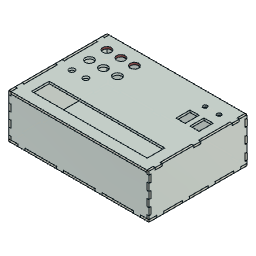
SimDash_Fusion (Autodesk Fusion 360 design; units mm, degrees)
Autodesk Fusion 360 part; units mm, degrees
(part 1 of 2)
sketch "Skizze1" plane through (0, 0, 0) normal (0, 0, 1) x (1, 0, 0)
  line L0 (-100, 70) -> (100, 70)
  line L1 (100, 70) -> (100, -70)
  line L2 (100, -70) -> (-100, -70)
  line L3 (-100, -70) -> (-100, 70)
  line L4 (-100, 70) -> (100, -70) construction
  line L5 (100, 70) -> (-100, -70) construction
  dimension "d1" = 200
  dimension "d2" = 140
  constraint horizontal L0
  constraint perpendicular L0 L1
  constraint parallel L0 L2
  constraint parallel L1 L3
  constraint coincident L4 origin
  constraint coincident L5 origin
  measures "d1" distance of L1.end L2.end
  measures "d2" distance of L0.end L1.end
extrude "Extrusion1" add sketch "Skizze1" along normal blind 3 makes body 1
sketch "Skizze2" plane through (0, 0, 3) normal (0, 0, 1) x (-1, 0, 0)
  line L0 (100, 70) -> (-100, 70)
  line L1 (-100, 70) -> (-100, -70)
  line L2 (-100, -70) -> (100, -70)
  line L3 (100, -70) -> (100, 70)
  line L4 (100, -70) -> (97, -70)
  line L5 (97, -70) -> (97, 70)
  line L6 (97, 70) -> (100, 70)
  line L7 (100, 70) -> (100, -70)
  dimension "d5" = 3
  constraint horizontal L4
  constraint vertical L5
  constraint horizontal L6
  constraint vertical L7
  constraint coincident L2.end L3.start
  measures "d5" distance of L2.end L4.end
extrude "Extrusion2" add sketch "Skizze2" along normal blind 60 separate body contours L0 L2 L3 L4 L5 L6 L7 picked at (99, 23.333333) makes body 2
sketch "Skizze3" plane through (0, 0, 3) normal (0, 0, -1) x (1, 0, 0)
  line L0 (-97, 70) -> (-100, 70)
  line L1 (-100, 70) -> (-100, -70)
  line L2 (-100, -70) -> (-97, -70)
  line L3 (-97, -70) -> (-97, 70)
  line L4 (-100, 60) -> (-97, 60)
  line L5 (-97, 60) -> (-97, 50)
  line L6 (-97, 50) -> (-100, 50)
  line L7 (-100, 50) -> (-100, 60)
  dimension "d8" = 3
  dimension "d9" = 10
  constraint horizontal L4
  constraint vertical L5
  constraint horizontal L6
  constraint vertical L7
  constraint coincident L1 L4.start
  measures "d8" distance of L4.start L4.end
  measures "d9" distance of L4.start L6.end
extrude "Extrusion3" add sketch "Skizze3" along normal blind 3 contours L1 L3 L4 L5 L6 L7 picked at (-99, 56.666667) bodies 2
pattern_linear "R-Anordnung1" count 4 spacing 36.666667 along (0, 1, 0) of "Extrusion3"
combine "Kombinieren1" operation cut target body 1 tool bodies 2 keep tools
sketch "Skizze4" plane through (0, 0, 3) normal (0, 0, 1) x (-1, 0, 0)
  line L0 (97, -60) -> (97, -50)
  line L1 (97, -50) -> (100, -50)
  line L2 (100, -50) -> (100, -23.333333)
  line L3 (100, -23.333333) -> (97, -23.333333)
  line L4 (97, -23.333333) -> (97, -13.333333)
  line L5 (97, -13.333333) -> (100, -13.333333)
  line L6 (100, -13.333333) -> (100, 13.333333)
  line L7 (100, 13.333333) -> (97, 13.333333)
  line L8 (97, 13.333333) -> (97, 23.333333)
  line L9 (97, 23.333333) -> (100, 23.333333)
  line L10 (100, 23.333333) -> (100, 50)
  line L11 (100, 50) -> (97, 50)
  line L12 (97, 50) -> (97, 60)
  line L13 (97, 60) -> (100, 60)
  line L14 (100, 60) -> (100, 70)
  line L15 (100, 70) -> (-100, 70)
  line L16 (-100, 70) -> (-100, -70)
  line L17 (-100, -70) -> (100, -70)
  line L18 (100, -70) -> (100, -60)
  line L19 (100, -60) -> (97, -60)
  line L20 (-100, -70) -> (-97, -70)
  line L21 (-97, -70) -> (-97, 70)
  line L22 (-97, 70) -> (-100, 70)
  line L23 (-100, 70) -> (-100, -70)
  dimension "d16" = 3
  constraint horizontal L20
  constraint vertical L21
  constraint horizontal L22
  constraint vertical L23
  constraint coincident L16.end L17.start
  measures "d16" distance of L16.end L20.end
sketch "Skizze6" plane through (0, 0, 3) normal (0, 0, 1) x (-1, 0, 0)
  line L0 (-100, -70) -> (100, -70)
  line L1 (100, -70) -> (100, -60)
  line L2 (100, -60) -> (97, -60)
  line L3 (97, -60) -> (97, -50)
  line L4 (97, -50) -> (100, -50)
  line L5 (100, -50) -> (100, -23.333333)
  line L6 (100, -23.333333) -> (97, -23.333333)
  line L7 (97, -23.333333) -> (97, -13.333333)
  line L8 (97, -13.333333) -> (100, -13.333333)
  line L9 (100, -13.333333) -> (100, 13.333333)
  line L10 (100, 13.333333) -> (97, 13.333333)
  line L11 (97, 13.333333) -> (97, 23.333333)
  line L12 (97, 23.333333) -> (100, 23.333333)
  line L13 (100, 23.333333) -> (100, 50)
  line L14 (100, 50) -> (97, 50)
  line L15 (97, 50) -> (97, 60)
  line L16 (97, 60) -> (100, 60)
  line L17 (100, 60) -> (100, 70)
  line L18 (100, 70) -> (-100, 70)
  line L19 (-100, 70) -> (-100, -70)
  line L20 (97.000041, -70) -> (-96.999959, -70)
  line L21 (-96.999959, -70) -> (-96.999959, -67)
  line L22 (-96.999959, -67) -> (97.000041, -67)
  line L23 (97.000041, -67) -> (97.000041, -70)
  dimension "d26" = 194
  dimension "d27" = 3
  constraint horizontal L20
  constraint vertical L21
  constraint horizontal L22
  constraint vertical L23
extrude "Extrusion6" add sketch "Skizze6" along normal blind 60 separate body contours L0 L20 L21 L22 L23 picked at (-32.333293, -68) makes body 3
sketch "Skizze7" plane through (96.999959, 0, 0) normal (1, 0, 0) x (0, 1, 0)
  line L0 (67, 3) -> (70, 3)
  line L1 (70, 3) -> (70, 63)
  line L2 (70, 63) -> (67, 63)
  line L3 (67, 63) -> (67, 3)
  line L4 (67, 58.682652) -> (70, 58.682652)
  line L5 (70, 58.682652) -> (70, 48.682652)
  line L6 (70, 48.682652) -> (67, 48.682652)
  line L7 (67, 48.682652) -> (67, 58.682652)
  dimension "d30" = 10
  constraint horizontal L4
  constraint vertical L5
  constraint horizontal L6
  constraint vertical L7
extrude "Extrusion7" add sketch "Skizze7" along normal blind 3.1 contours L1 L3 L4 L5 L6 L7 picked at (68, 55.349319) bodies 3
pattern_linear "R-Anordnung3" count 3 spacing 21 along (0, 0, -1) of "Extrusion7"
sketch "Skizze10" plane through (-97.000041, 0, 0) normal (-1, 0, 0) x (0, -1, 0)
  line L0 (-70, 3) -> (-67, 3)
  line L1 (-67, 3) -> (-67, 63)
  line L2 (-67, 63) -> (-70, 63)
  line L3 (-70, 63) -> (-70, 3)
  line L4 (-70, 58.048511) -> (-67, 58.048511)
  line L5 (-67, 58.048511) -> (-67, 48.048511)
  line L6 (-67, 48.048511) -> (-70, 48.048511)
  line L7 (-70, 48.048511) -> (-70, 58.048511)
  dimension "d43" = 10
  constraint horizontal L4
  constraint vertical L5
  constraint horizontal L6
  constraint vertical L7
extrude "Extrusion10" add sketch "Skizze10" along normal blind 3 contours L1 L3 L4 L5 L6 L7 picked at (-69, 54.715177) bodies 3
pattern_linear "R-Anordnung4" count 3 spacing 20 along (0, 0, -1) of "Extrusion10"
sketch "Skizze11" plane through (0, 0, 3) normal (0, 0, -1) x (1, 0, 0)
  line L0 (96.999959, -67) -> (-97.000041, -67)
  line L1 (-97.000041, -67) -> (-97.000041, -70)
  line L2 (-97.000041, -70) -> (96.999959, -70)
  line L3 (96.999959, -70) -> (96.999959, -67)
  line L4 (-90.254959, -67) -> (-80.254959, -67)
  line L5 (-80.254959, -67) -> (-80.254959, -70)
  line L6 (-80.254959, -70) -> (-90.254959, -70)
  line L7 (-90.254959, -70) -> (-90.254959, -67)
  dimension "d50" = 10
  constraint horizontal L4
  constraint vertical L5
  constraint horizontal L6
  constraint vertical L7
extrude "Extrusion11" add sketch "Skizze11" along normal blind 3 contours L0 L2 L4 L5 L6 L7 picked at (-86.921626, -68) bodies 3
pattern_linear "R-Anordnung5" count 4 spacing 56.666667 along (1, 0, 0) of "Extrusion11"
combine "Kombinieren3" operation cut target body 2 tool bodies 3 keep tools
combine "Kombinieren4" operation cut target body 1 tool bodies 3 keep tools
sketch "Skizze12" plane through (0, 0, 3) normal (0, 0, 1) x (-1, 0, 0)
  line L0 (-100, -70) -> (-89.745041, -70)
  line L1 (-89.745041, -70) -> (-89.745041, -67)
  line L2 (-89.745041, -67) -> (-79.745041, -67)
  line L3 (-79.745041, -67) -> (-79.745041, -70)
  line L4 (-79.745041, -70) -> (-33.078374, -70)
  line L5 (-33.078374, -70) -> (-33.078374, -67)
  line L6 (-33.078374, -67) -> (-23.078374, -67)
  line L7 (-23.078374, -67) -> (-23.078374, -70)
  line L8 (-23.078374, -70) -> (23.588293, -70)
  line L9 (23.588293, -70) -> (23.588293, -67)
  line L10 (23.588293, -67) -> (33.588293, -67)
  line L11 (33.588293, -67) -> (33.588293, -70)
  line L12 (33.588293, -70) -> (80.254959, -70)
  line L13 (80.254959, -70) -> (80.254959, -67)
  line L14 (80.254959, -67) -> (90.254959, -67)
  line L15 (90.254959, -67) -> (90.254959, -70)
  line L16 (90.254959, -70) -> (100, -70)
  line L17 (100, -70) -> (100, -60)
  line L18 (100, -60) -> (97, -60)
  line L19 (97, -60) -> (97, -50)
  line L20 (97, -50) -> (100, -50)
  line L21 (100, -50) -> (100, -23.333333)
  line L22 (100, -23.333333) -> (97, -23.333333)
  line L23 (97, -23.333333) -> (97, -13.333333)
  line L24 (97, -13.333333) -> (100, -13.333333)
  line L25 (100, -13.333333) -> (100, 13.333333)
  line L26 (100, 13.333333) -> (97, 13.333333)
  line L27 (97, 13.333333) -> (97, 23.333333)
  line L28 (97, 23.333333) -> (100, 23.333333)
  line L29 (100, 23.333333) -> (100, 50)
  line L30 (100, 50) -> (97, 50)
  line L31 (97, 50) -> (97, 60)
  line L32 (97, 60) -> (100, 60)
  line L33 (100, 60) -> (100, 70)
  line L34 (100, 70) -> (-100, 70)
  line L35 (-100, 70) -> (-100, -70)
  line L36 (-100, -70) -> (-97, -70)
  line L37 (-97, -70) -> (-97, 70)
  line L38 (-97, 70) -> (-100, 70)
  line L39 (-100, 70) -> (-100, -70)
  dimension "d59" = 3
  constraint horizontal L36
  constraint vertical L37
  constraint horizontal L38
  constraint vertical L39
  constraint coincident L0.start L35.end
  measures "d59" distance of L0.start L36.end
extrude "Extrusion13" add sketch "Skizze12" along normal blind 60 separate body contours L0 L34 L35 L36 L37 L38 L39 picked at (-99, 23.333333) makes body 4
combine "Kombinieren5" operation cut target body 4 tool bodies 3 keep tools
combine "Kombinieren6" operation cut target body 4 tool bodies 3 keep tools
sketch "Skizze13" plane through (0, 0, 3) normal (0, 0, -1) x (1, 0, 0)
  line L0 (100, -70) -> (100, 70)
  line L1 (100, 70) -> (97, 70)
  line L2 (97, 70) -> (97, -70)
  line L3 (97, -70) -> (100, -70)
  line L4 (97, 58.902439) -> (100, 58.902439)
  line L5 (100, 58.902439) -> (100, 48.902439)
  line L6 (100, 48.902439) -> (97, 48.902439)
  line L7 (97, 48.902439) -> (97, 58.902439)
  dimension "d62" = 10
  constraint horizontal L4
  constraint vertical L5
  constraint horizontal L6
  constraint vertical L7
extrude "Extrusion14" add sketch "Skizze13" along normal blind 3 contours L0 L2 L4 L5 L6 L7 picked at (99, 52.235772) bodies 4
pattern_linear "R-Anordnung6" count 4 spacing 36.666667 along (0, 1, 0) of "Extrusion14"
combine "Kombinieren7" operation cut target body 1 tool bodies 4 keep tools
sketch "Skizze14" plane through (0, 0, 3) normal (0, 0, 1) x (-1, 0, 0)
  line L0 (-97, 58.902439) -> (-97, 48.902439)
  line L1 (-97, 48.902439) -> (-100, 48.902439)
  line L2 (-100, 48.902439) -> (-100, 22.235772)
  line L3 (-100, 22.235772) -> (-97, 22.235772)
  line L4 (-97, 22.235772) -> (-97, 12.235772)
  line L5 (-97, 12.235772) -> (-100, 12.235772)
  line L6 (-100, 12.235772) -> (-100, -14.430895)
  line L7 (-100, -14.430895) -> (-97, -14.430895)
  line L8 (-97, -14.430895) -> (-97, -24.430895)
  line L9 (-97, -24.430895) -> (-100, -24.430895)
  line L10 (-100, -24.430895) -> (-100, -51.097561)
  line L11 (-100, -51.097561) -> (-97, -51.097561)
  line L12 (-97, -51.097561) -> (-97, -61.097561)
  line L13 (-97, -61.097561) -> (-100, -61.097561)
  line L14 (-100, -61.097561) -> (-100, -70)
  line L15 (-100, -70) -> (-89.745041, -70)
  line L16 (-89.745041, -70) -> (-89.745041, -67)
  line L17 (-89.745041, -67) -> (-79.745041, -67)
  line L18 (-79.745041, -67) -> (-79.745041, -70)
  line L19 (-79.745041, -70) -> (-33.078374, -70)
  line L20 (-33.078374, -70) -> (-33.078374, -67)
  line L21 (-33.078374, -67) -> (-23.078374, -67)
  line L22 (-23.078374, -67) -> (-23.078374, -70)
  line L23 (-23.078374, -70) -> (23.588293, -70)
  line L24 (23.588293, -70) -> (23.588293, -67)
  line L25 (23.588293, -67) -> (33.588293, -67)
  line L26 (33.588293, -67) -> (33.588293, -70)
  line L27 (33.588293, -70) -> (80.254959, -70)
  line L28 (80.254959, -70) -> (80.254959, -67)
  line L29 (80.254959, -67) -> (90.254959, -67)
  line L30 (90.254959, -67) -> (90.254959, -70)
  line L31 (90.254959, -70) -> (100, -70)
  line L32 (100, -70) -> (100, -60)
  line L33 (100, -60) -> (97, -60)
  line L34 (97, -60) -> (97, -50)
  line L35 (97, -50) -> (100, -50)
  line L36 (100, -50) -> (100, -23.333333)
  line L37 (100, -23.333333) -> (97, -23.333333)
  line L38 (97, -23.333333) -> (97, -13.333333)
  line L39 (97, -13.333333) -> (100, -13.333333)
  line L40 (100, -13.333333) -> (100, 13.333333)
  line L41 (100, 13.333333) -> (97, 13.333333)
  line L42 (97, 13.333333) -> (97, 23.333333)
  line L43 (97, 23.333333) -> (100, 23.333333)
  line L44 (100, 23.333333) -> (100, 50)
  line L45 (100, 50) -> (97, 50)
  line L46 (97, 50) -> (97, 60)
  line L47 (97, 60) -> (100, 60)
  line L48 (100, 60) -> (100, 70)
  line L49 (100, 70) -> (-100, 70)
  line L50 (-100, 70) -> (-100, 58.902439)
  line L51 (-100, 58.902439) -> (-97, 58.902439)
  line L52 (97, 70) -> (-97.000001, 70)
  line L53 (-97.000001, 70) -> (-97.000001, 67)
  line L54 (-97.000001, 67) -> (97, 67)
  line L55 (97, 67) -> (97, 70)
  dimension "d69" = 3
  constraint horizontal L52
  constraint vertical L53
  constraint horizontal L54
  constraint vertical L55
  constraint coincident L49 L52.start
  measures "d69" distance of L52.start L54.end
extrude "Extrusion15" add sketch "Skizze14" along normal blind 60 separate body contours L49 L52 L53 L54 L55 picked at (-32.333334, 69) makes body 5
sketch "Skizze15" plane through (-97, 0, 0) normal (-1, 0, 0) x (0, -1, 0)
  line L0 (67, 3) -> (70, 3)
  line L1 (70, 3) -> (70, 63)
  line L2 (70, 63) -> (67, 63)
  line L3 (67, 63) -> (67, 3)
  line L4 (67, 57.564108) -> (70, 57.564108)
  line L5 (70, 57.564108) -> (70, 47.564108)
  line L6 (70, 47.564108) -> (67, 47.564108)
  line L7 (67, 47.564108) -> (67, 57.564108)
  dimension "d72" = 10
  constraint horizontal L4
  constraint vertical L5
  constraint horizontal L6
  constraint vertical L7
extrude "Extrusion16" add sketch "Skizze15" along normal blind 3 contours L1 L3 L4 L5 L6 L7 picked at (68, 54.230775) bodies 5
pattern_linear "R-Anordnung7" count 3 spacing 20 along (0, 0, -1) of "Extrusion16"
combine "Kombinieren8" operation cut target body 2 tool bodies 5 keep tools
sketch "Skizze16" plane through (0, 0, 3) normal (0, 0, -1) x (1, 0, 0)
  line L0 (-97, 70) -> (-97, 67)
  line L1 (-97, 67) -> (97.000001, 67)
  line L2 (97.000001, 67) -> (97.000001, 70)
  line L3 (97.000001, 70) -> (-97, 70)
  line L4 (-86.937173, 70) -> (-76.937173, 70)
  line L5 (-76.937173, 70) -> (-76.937173, 67)
  line L6 (-76.937173, 67) -> (-86.937173, 67)
  line L7 (-86.937173, 67) -> (-86.937173, 70)
  dimension "d79" = 10
  constraint horizontal L4
  constraint vertical L5
  constraint horizontal L6
  constraint vertical L7
extrude "Extrusion17" add sketch "Skizze16" along normal blind 3 contours L1 L3 L4 L5 L6 L7 picked at (-83.60384, 69) bodies 5
pattern_linear "R-Anordnung8" count 4 spacing 55 along (1, 0, 0) of "Extrusion17"
combine "Kombinieren9" operation cut target body 1 tool bodies 5 keep tools
sketch "Skizze17" plane through (97.000001, 0, 0) normal (1, 0, 0) x (0, 1, 0)
  line L0 (-70, 3) -> (-67, 3)
  line L1 (-67, 3) -> (-67, 63)
  line L2 (-67, 63) -> (-70, 63)
  line L3 (-70, 63) -> (-70, 3)
  line L4 (-70, 57.960939) -> (-67, 57.960939)
  line L5 (-67, 57.960939) -> (-67, 47.960939)
  line L6 (-67, 47.960939) -> (-70, 47.960939)
  line L7 (-70, 47.960939) -> (-70, 57.960939)
  dimension "d86" = 10
  constraint horizontal L4
  constraint vertical L5
  constraint horizontal L6
  constraint vertical L7
extrude "Extrusion18" add sketch "Skizze17" along normal blind 3 contours L1 L3 L4 L5 L6 L7 picked at (-69, 54.627606) bodies 5
pattern_linear "R-Anordnung9" count 3 spacing 20 along (0, 0, -1) of "Extrusion18"
combine "Kombinieren10" operation cut target body 4 tool bodies 5 keep tools
sketch "Skizze18" plane through (97, 0, 0) normal (-1, 0, 0) x (0, -1, 0)
  line L0 (67, 7.960939) -> (67, 17.960939)
  line L1 (67, 17.960939) -> (70, 17.960939)
  line L2 (70, 17.960939) -> (70, 27.960939)
  line L3 (70, 27.960939) -> (67, 27.960939)
  line L4 (67, 27.960939) -> (67, 37.960939)
  line L5 (67, 37.960939) -> (70, 37.960939)
  line L6 (70, 37.960939) -> (70, 47.960939)
  line L7 (70, 47.960939) -> (67, 47.960939)
  line L8 (67, 47.960939) -> (67, 57.960939)
  line L9 (67, 57.960939) -> (70, 57.960939)
  line L10 (70, 57.960939) -> (70, 63)
  line L11 (70, 63) -> (-70, 63)
  line L12 (-70, 63) -> (-70, 58.682652)
  line L13 (-70, 58.682652) -> (-67, 58.682652)
  line L14 (-67, 58.682652) -> (-67, 48.682652)
  line L15 (-67, 48.682652) -> (-70, 48.682652)
  line L16 (-70, 48.682652) -> (-70, 37.682652)
  line L17 (-70, 37.682652) -> (-67, 37.682652)
  line L18 (-67, 37.682652) -> (-67, 27.682652)
  line L19 (-67, 27.682652) -> (-70, 27.682652)
  line L20 (-70, 27.682652) -> (-70, 16.682652)
  line L21 (-70, 16.682652) -> (-67, 16.682652)
  line L22 (-67, 16.682652) -> (-67, 6.682652)
  line L23 (-67, 6.682652) -> (-70, 6.682652)
  line L24 (-70, 6.682652) -> (-70, 3)
  line L25 (-70, 3) -> (-61.097561, 3)
  line L26 (-61.097561, 3) -> (-61.097561, 0)
  line L27 (-61.097561, 0) -> (-51.097561, 0)
  line L28 (-51.097561, 0) -> (-51.097561, 3)
  line L29 (-51.097561, 3) -> (-24.430895, 3)
  line L30 (-24.430895, 3) -> (-24.430895, 0)
  line L31 (-24.430895, 0) -> (-14.430895, 0)
  line L32 (-14.430895, 0) -> (-14.430895, 3)
  line L33 (-14.430895, 3) -> (12.235772, 3)
  line L34 (12.235772, 3) -> (12.235772, 0)
  line L35 (12.235772, 0) -> (22.235772, 0)
  line L36 (22.235772, 0) -> (22.235772, 3)
  line L37 (22.235772, 3) -> (48.902439, 3)
  line L38 (48.902439, 3) -> (48.902439, 0)
  line L39 (48.902439, 0) -> (58.902439, 0)
  line L40 (58.902439, 0) -> (58.902439, 3)
  line L41 (58.902439, 3) -> (70, 3)
  line L42 (70, 3) -> (70, 7.960939)
  line L43 (70, 7.960939) -> (67, 7.960939)
  line L44 (-70, 63) -> (70, 63)
  line L45 (70, 63) -> (70, 60)
  line L46 (70, 60) -> (-70, 60)
  line L47 (-70, 60) -> (-70, 63)
  dimension "d93" = 3
  constraint horizontal L44
  constraint vertical L45
  constraint horizontal L46
  constraint vertical L47
  constraint coincident L11.end L12.start
  measures "d93" distance of L11.end L46.end
extrude "Extrusion19" add sketch "Skizze18" along normal blind 194 separate body contours L10 L11 L12 L44 L45 L46 L47 picked at (23.333333, 61) makes body 6
sketch "Skizze19" plane through (-97, 0, 0) normal (-1, 0, 0) x (0, -1, 0)
  line L0 (-70, 60) -> (70, 60)
  line L1 (70, 60) -> (70, 63)
  line L2 (70, 63) -> (-70, 63)
  line L3 (-70, 63) -> (-70, 60)
  line L4 (-63.742894, 63) -> (-53.742894, 63)
  line L5 (-53.742894, 63) -> (-53.742894, 60)
  line L6 (-53.742894, 60) -> (-63.742894, 60)
  line L7 (-63.742894, 60) -> (-63.742894, 63)
  dimension "d96" = 10
  constraint horizontal L4
  constraint vertical L5
  constraint horizontal L6
  constraint vertical L7
extrude "Extrusion20" add sketch "Skizze19" along normal blind 3 contours L0 L2 L4 L5 L6 L7 picked at (-60.409561, 61) bodies 6
pattern_linear "R-Anordnung10" count 3 spacing 57.5 along (0, -1, 0) of "Extrusion20"
combine "Kombinieren11" operation cut target body 2 tool bodies 6 keep tools
sketch "Skizze20" plane through (97, 0, 0) normal (1, 0, 0) x (0, 1, 0)
  line L0 (-70, 60) -> (70, 60)
  line L1 (70, 60) -> (70, 63)
  line L2 (70, 63) -> (-70, 63)
  line L3 (-70, 63) -> (-70, 60)
  line L4 (-61.18405, 63) -> (-51.18405, 63)
  line L5 (-51.18405, 63) -> (-51.18405, 60)
  line L6 (-51.18405, 60) -> (-61.18405, 60)
  line L7 (-61.18405, 60) -> (-61.18405, 63)
  dimension "d103" = 10
  constraint horizontal L4
  constraint vertical L5
  constraint horizontal L6
  constraint vertical L7
extrude "Extrusion21" add sketch "Skizze20" along normal blind 3 contours L0 L2 L4 L5 L6 L7 picked at (-57.850717, 62) bodies 6
pattern_linear "R-Anordnung11" count 3 spacing 55 along (0, 1, 0) of "Extrusion21"
combine "Kombinieren12" operation cut target body 4 tool bodies 6 keep tools
combine "Kombinieren13" operation cut target body 5 tool bodies 6 keep tools
combine "Kombinieren14" operation cut target body 3 tool bodies 6 keep tools
sketch "Skizze23" plane through (0, 0, 63) normal (0, 0, 1) x (-1, 0, 0)
  line L0 (-97, -48.81595) -> (-100, -48.81595)
  line L1 (-100, -48.81595) -> (-100, -58.81595)
  line L2 (-100, -58.81595) -> (-97, -58.81595)
  line L3 (-97, -58.81595) -> (-97, -70)
  line L4 (-97, -70) -> (97, -70)
  line L5 (97, -70) -> (97, -63.742894)
  line L6 (97, -63.742894) -> (100, -63.742894)
  line L7 (100, -63.742894) -> (100, -53.742894)
  line L8 (100, -53.742894) -> (97, -53.742894)
  line L9 (97, -53.742894) -> (97, -6.242894)
  line L10 (97, -6.242894) -> (100, -6.242894)
  line L11 (100, -6.242894) -> (100, 3.757106)
  line L12 (100, 3.757106) -> (97, 3.757106)
  line L13 (97, 3.757106) -> (97, 51.257106)
  line L14 (97, 51.257106) -> (100, 51.257106)
  line L15 (100, 51.257106) -> (100, 61.257106)
  line L16 (100, 61.257106) -> (97, 61.257106)
  line L17 (97, 61.257106) -> (97, 70)
  line L18 (97, 70) -> (-97, 70)
  line L19 (-97, 70) -> (-97, 61.18405)
  line L20 (-97, 61.18405) -> (-100, 61.18405)
  line L21 (-100, 61.18405) -> (-100, 51.18405)
  line L22 (-100, 51.18405) -> (-97, 51.18405)
  line L23 (-97, 51.18405) -> (-97, 6.18405)
  line L24 (-97, 6.18405) -> (-100, 6.18405)
  line L25 (-100, 6.18405) -> (-100, -3.81595)
  line L26 (-100, -3.81595) -> (-97, -3.81595)
  line L27 (-97, -3.81595) -> (-97, -48.81595)
  circle A0 centre (80, -50) radius 6
  circle A1 centre (60, -50) radius 6
  circle A2 centre (40.782868, -50.075086) radius 6
  dimension "d124" = 12
  dimension "d125" = 12
  dimension "d126" = 12
  measures "d124" diameter of A0
  measures "d125" diameter of A1
  measures "d126" diameter of A2
extrude "Extrusion24" cut sketch "Skizze23" against normal blind 10 contours A0 | A1 | A2 picked at (79.119858, -46.143845) picked at (61.921795, -48.743663) picked at (40.633408, -48.345998) bodies 6
sketch "Skizze24" plane through (0, 0, 63) normal (0, 0, 1) x (-1, 0, 0)
  circle A0 centre (80, -50) radius 6
  circle A1 centre (60, -50) radius 6
  circle A2 centre (40.782868, -50.075086) radius 6
  line L0 (-97, -48.81595) -> (-100, -48.81595)
  line L1 (-100, -48.81595) -> (-100, -58.81595)
  line L2 (-100, -58.81595) -> (-97, -58.81595)
  line L3 (-97, -58.81595) -> (-97, -70)
  line L4 (-97, -70) -> (97, -70)
  line L5 (97, -70) -> (97, -63.742894)
  line L6 (97, -63.742894) -> (100, -63.742894)
  line L7 (100, -63.742894) -> (100, -53.742894)
  line L8 (100, -53.742894) -> (97, -53.742894)
  line L9 (97, -53.742894) -> (97, -6.242894)
  line L10 (97, -6.242894) -> (100, -6.242894)
  line L11 (100, -6.242894) -> (100, 3.757106)
  line L12 (100, 3.757106) -> (97, 3.757106)
  line L13 (97, 3.757106) -> (97, 51.257106)
  line L14 (97, 51.257106) -> (100, 51.257106)
  line L15 (100, 51.257106) -> (100, 61.257106)
  line L16 (100, 61.257106) -> (97, 61.257106)
  line L17 (97, 61.257106) -> (97, 70)
  line L18 (97, 70) -> (-97, 70)
  line L19 (-97, 70) -> (-97, 61.18405)
  line L20 (-97, 61.18405) -> (-100, 61.18405)
  line L21 (-100, 61.18405) -> (-100, 51.18405)
  line L22 (-100, 51.18405) -> (-97, 51.18405)
  line L23 (-97, 51.18405) -> (-97, 6.18405)
  line L24 (-97, 6.18405) -> (-100, 6.18405)
  line L25 (-100, 6.18405) -> (-100, -3.81595)
  line L26 (-100, -3.81595) -> (-97, -3.81595)
  line L27 (-97, -3.81595) -> (-97, -48.81595)
  circle A3 centre (-80, -50) radius 3
  circle A4 centre (-60, -50) radius 3
  dimension "d129" = 6
  dimension "d130" = 6
  measures "d129" diameter of A3
  measures "d130" diameter of A4
extrude "Extrusion25" cut sketch "Skizze24" against normal blind 20 contours A3 | A4 picked at (-79.179086, -49.034986) picked at (-60.57473, -48.136771) bodies 6
sketch "Skizze25" plane through (0, 0, 63) normal (0, 0, 1) x (-1, 0, 0)
  circle A0 centre (-60, -50) radius 3
  circle A1 centre (-80, -50) radius 3
  circle A2 centre (80, -50) radius 6
  circle A3 centre (60, -50) radius 6
  circle A4 centre (40.782868, -50.075086) radius 6
  line L0 (-97, -48.81595) -> (-100, -48.81595)
  line L1 (-100, -48.81595) -> (-100, -58.81595)
  line L2 (-100, -58.81595) -> (-97, -58.81595)
  line L3 (-97, -58.81595) -> (-97, -70)
  line L4 (-97, -70) -> (97, -70)
  line L5 (97, -70) -> (97, -63.742894)
  line L6 (97, -63.742894) -> (100, -63.742894)
  line L7 (100, -63.742894) -> (100, -53.742894)
  line L8 (100, -53.742894) -> (97, -53.742894)
  line L9 (97, -53.742894) -> (97, -6.242894)
  line L10 (97, -6.242894) -> (100, -6.242894)
  line L11 (100, -6.242894) -> (100, 3.757106)
  line L12 (100, 3.757106) -> (97, 3.757106)
  line L13 (97, 3.757106) -> (97, 51.257106)
  line L14 (97, 51.257106) -> (100, 51.257106)
  line L15 (100, 51.257106) -> (100, 61.257106)
  line L16 (100, 61.257106) -> (97, 61.257106)
  line L17 (97, 61.257106) -> (97, 70)
  line L18 (97, 70) -> (-97, 70)
  line L19 (-97, 70) -> (-97, 61.18405)
  line L20 (-97, 61.18405) -> (-100, 61.18405)
  line L21 (-100, 61.18405) -> (-100, 51.18405)
  line L22 (-100, 51.18405) -> (-97, 51.18405)
  line L23 (-97, 51.18405) -> (-97, 6.18405)
  line L24 (-97, 6.18405) -> (-100, 6.18405)
  line L25 (-100, 6.18405) -> (-100, -3.81595)
  line L26 (-100, -3.81595) -> (-97, -3.81595)
  line L27 (-97, -3.81595) -> (-97, -48.81595)
  line L28 (-73.409655, -35.161049) -> (-86.409655, -35.161049)
  line L29 (-86.409655, -35.161049) -> (-86.409655, -15.161049)
  line L30 (-86.409655, -15.161049) -> (-73.409655, -15.161049)
  line L31 (-73.409655, -15.161049) -> (-73.409655, -35.161049)
  line L32 (-73.409655, -35.161049) -> (-86.409655, -15.161049) construction
  line L33 (-86.409655, -35.161049) -> (-73.409655, -15.161049) construction
  line L34 (-53.616861, -35.006887) -> (-66.616861, -35.006887)
  line L35 (-66.616861, -35.006887) -> (-66.616861, -15.006887)
  line L36 (-66.616861, -15.006887) -> (-53.616861, -15.006887)
  line L37 (-53.616861, -15.006887) -> (-53.616861, -35.006887)
  line L38 (-53.616861, -35.006887) -> (-66.616861, -15.006887) construction
  line L39 (-66.616861, -35.006887) -> (-53.616861, -15.006887) construction
  point P0 (-79.909655, -25.161049)
  point P1 (-60.116861, -25.006887)
  dimension "d133" = 13
  dimension "d134" = 20
  dimension "d135" = 13
  constraint horizontal L28
  constraint perpendicular L28 L29
  constraint parallel L28 L30
  constraint parallel L29 L31
  constraint horizontal L34
  constraint perpendicular L34 L35
  constraint parallel L34 L36
  constraint parallel L35 L37
extrude "Extrusion26" cut sketch "Skizze25" against normal blind 25 contours L28 L29 L30 L31 | L34 L35 L36 L37 picked at (-82.076322, -28.494382) picked at (-62.283528, -21.673554) bodies 6
sketch "Skizze26" plane through (0, 0, 63) normal (0, 0, 1) x (-1, 0, 0)
  line L0 (-66.616861, -35.006887) -> (-66.616861, -15.006887)
  line L1 (-66.616861, -15.006887) -> (-53.616861, -15.006887)
  line L2 (-53.616861, -15.006887) -> (-53.616861, -35.006887)
  line L3 (-53.616861, -35.006887) -> (-66.616861, -35.006887)
  line L4 (-86.409655, -35.161049) -> (-86.409655, -15.161049)
  line L5 (-86.409655, -15.161049) -> (-73.409655, -15.161049)
  line L6 (-73.409655, -15.161049) -> (-73.409655, -35.161049)
  line L7 (-73.409655, -35.161049) -> (-86.409655, -35.161049)
  circle A0 centre (-60, -50) radius 3
  circle A1 centre (-80, -50) radius 3
  circle A2 centre (80, -50) radius 6
  circle A3 centre (60, -50) radius 6
  circle A4 centre (40.782868, -50.075086) radius 6
  line L8 (-97, -48.81595) -> (-100, -48.81595)
  line L9 (-100, -48.81595) -> (-100, -58.81595)
  line L10 (-100, -58.81595) -> (-97, -58.81595)
  line L11 (-97, -58.81595) -> (-97, -70)
  line L12 (-97, -70) -> (97, -70)
  line L13 (97, -70) -> (97, -63.742894)
  line L14 (97, -63.742894) -> (100, -63.742894)
  line L15 (100, -63.742894) -> (100, -53.742894)
  line L16 (100, -53.742894) -> (97, -53.742894)
  line L17 (97, -53.742894) -> (97, -6.242894)
  line L18 (97, -6.242894) -> (100, -6.242894)
  line L19 (100, -6.242894) -> (100, 3.757106)
  line L20 (100, 3.757106) -> (97, 3.757106)
  line L21 (97, 3.757106) -> (97, 51.257106)
  line L22 (97, 51.257106) -> (100, 51.257106)
  line L23 (100, 51.257106) -> (100, 61.257106)
  line L24 (100, 61.257106) -> (97, 61.257106)
  line L25 (97, 61.257106) -> (97, 70)
  line L26 (97, 70) -> (-97, 70)
  line L27 (-97, 70) -> (-97, 61.18405)
  line L28 (-97, 61.18405) -> (-100, 61.18405)
  line L29 (-100, 61.18405) -> (-100, 51.18405)
  line L30 (-100, 51.18405) -> (-97, 51.18405)
  line L31 (-97, 51.18405) -> (-97, 6.18405)
  line L32 (-97, 6.18405) -> (-100, 6.18405)
  line L33 (-100, 6.18405) -> (-100, -3.81595)
  line L34 (-100, -3.81595) -> (-97, -3.81595)
  line L35 (-97, -3.81595) -> (-97, -48.81595)
  circle A5 centre (80, -25) radius 6
  circle A6 centre (60, -25) radius 6
  circle A7 centre (40, -25) radius 6
  dimension "d138" = 12
  dimension "d139" = 12
  dimension "d140" = 12
  measures "d138" diameter of A5
  measures "d139" diameter of A6
  measures "d140" diameter of A7
extrude "Extrusion27" cut sketch "Skizze26" against normal blind 12 contours A5 | A6 | A7 picked at (80.581222, -21.143845) picked at (57.46738, -26.2593) picked at (41.581222, -26.864711) bodies 6
sketch "Skizze27" plane through (0, 0, 63) normal (0, 0, 1) x (-1, 0, 0)
  circle A0 centre (60, -25) radius 6
  circle A1 centre (40, -25) radius 6
  circle A2 centre (80, -25) radius 6
  line L0 (-66.616861, -35.006887) -> (-66.616861, -15.006887)
  line L1 (-66.616861, -15.006887) -> (-53.616861, -15.006887)
  line L2 (-53.616861, -15.006887) -> (-53.616861, -35.006887)
  line L3 (-53.616861, -35.006887) -> (-66.616861, -35.006887)
  line L4 (-86.409655, -35.161049) -> (-86.409655, -15.161049)
  line L5 (-86.409655, -15.161049) -> (-73.409655, -15.161049)
  line L6 (-73.409655, -15.161049) -> (-73.409655, -35.161049)
  line L7 (-73.409655, -35.161049) -> (-86.409655, -35.161049)
  circle A3 centre (-60, -50) radius 3
  circle A4 centre (-80, -50) radius 3
  circle A5 centre (80, -50) radius 6
  circle A6 centre (60, -50) radius 6
  circle A7 centre (40.782868, -50.075086) radius 6
  line L8 (-97, -48.81595) -> (-100, -48.81595)
  line L9 (-100, -48.81595) -> (-100, -58.81595)
  line L10 (-100, -58.81595) -> (-97, -58.81595)
  line L11 (-97, -58.81595) -> (-97, -70)
  line L12 (-97, -70) -> (97, -70)
  line L13 (97, -70) -> (97, -63.742894)
  line L14 (97, -63.742894) -> (100, -63.742894)
  line L15 (100, -63.742894) -> (100, -53.742894)
  line L16 (100, -53.742894) -> (97, -53.742894)
  line L17 (97, -53.742894) -> (97, -6.242894)
  line L18 (97, -6.242894) -> (100, -6.242894)
  line L19 (100, -6.242894) -> (100, 3.757106)
  line L20 (100, 3.757106) -> (97, 3.757106)
  line L21 (97, 3.757106) -> (97, 51.257106)
  line L22 (97, 51.257106) -> (100, 51.257106)
  line L23 (100, 51.257106) -> (100, 61.257106)
  line L24 (100, 61.257106) -> (97, 61.257106)
  line L25 (97, 61.257106) -> (97, 70)
  line L26 (97, 70) -> (-97, 70)
  line L27 (-97, 70) -> (-97, 61.18405)
  line L28 (-97, 61.18405) -> (-100, 61.18405)
  line L29 (-100, 61.18405) -> (-100, 51.18405)
  line L30 (-100, 51.18405) -> (-97, 51.18405)
  line L31 (-97, 51.18405) -> (-97, 6.18405)
  line L32 (-97, 6.18405) -> (-100, 6.18405)
  line L33 (-100, 6.18405) -> (-100, -3.81595)
  line L34 (-100, -3.81595) -> (-97, -3.81595)
  line L35 (-97, -3.81595) -> (-97, -48.81595)
  circle A8 centre (80, 0) radius 4
  circle A9 centre (60, 0) radius 4
  dimension "d143" = 8
  dimension "d144" = 8
  measures "d143" diameter of A8
  measures "d144" diameter of A9
extrude "Extrusion28" cut sketch "Skizze27" against normal blind 12 contours A8 | A9 picked at (78.926117, 1.329605) picked at (58.770247, -0.198723) bodies 6
sketch "Skizze28" plane through (0, 0, 63) normal (0, 0, 1) x (-1, 0, 0)
  circle A0 centre (80, 0) radius 4
  circle A1 centre (60, 0) radius 4
  circle A2 centre (60, -25) radius 6
  circle A3 centre (40, -25) radius 6
  circle A4 centre (80, -25) radius 6
  line L0 (-66.616861, -35.006887) -> (-66.616861, -15.006887)
  line L1 (-66.616861, -15.006887) -> (-53.616861, -15.006887)
  line L2 (-53.616861, -15.006887) -> (-53.616861, -35.006887)
  line L3 (-53.616861, -35.006887) -> (-66.616861, -35.006887)
  line L4 (-86.409655, -35.161049) -> (-86.409655, -15.161049)
  line L5 (-86.409655, -15.161049) -> (-73.409655, -15.161049)
  line L6 (-73.409655, -15.161049) -> (-73.409655, -35.161049)
  line L7 (-73.409655, -35.161049) -> (-86.409655, -35.161049)
  circle A5 centre (-60, -50) radius 3
  circle A6 centre (-80, -50) radius 3
  circle A7 centre (80, -50) radius 6
  circle A8 centre (60, -50) radius 6
  circle A9 centre (40.782868, -50.075086) radius 6
  line L8 (-97, -48.81595) -> (-100, -48.81595)
  line L9 (-100, -48.81595) -> (-100, -58.81595)
  line L10 (-100, -58.81595) -> (-97, -58.81595)
  line L11 (-97, -58.81595) -> (-97, -70)
  line L12 (-97, -70) -> (97, -70)
  line L13 (97, -70) -> (97, -63.742894)
  line L14 (97, -63.742894) -> (100, -63.742894)
  line L15 (100, -63.742894) -> (100, -53.742894)
  line L16 (100, -53.742894) -> (97, -53.742894)
  line L17 (97, -53.742894) -> (97, -6.242894)
  line L18 (97, -6.242894) -> (100, -6.242894)
  line L19 (100, -6.242894) -> (100, 3.757106)
  line L20 (100, 3.757106) -> (97, 3.757106)
  line L21 (97, 3.757106) -> (97, 51.257106)
  line L22 (97, 51.257106) -> (100, 51.257106)
  line L23 (100, 51.257106) -> (100, 61.257106)
  line L24 (100, 61.257106) -> (97, 61.257106)
  line L25 (97, 61.257106) -> (97, 70)
  line L26 (97, 70) -> (-97, 70)
  line L27 (-97, 70) -> (-97, 61.18405)
  line L28 (-97, 61.18405) -> (-100, 61.18405)
  line L29 (-100, 61.18405) -> (-100, 51.18405)
  line L30 (-100, 51.18405) -> (-97, 51.18405)
  line L31 (-97, 51.18405) -> (-97, 6.18405)
  line L32 (-97, 6.18405) -> (-100, 6.18405)
  line L33 (-100, 6.18405) -> (-100, -3.81595)
  line L34 (-100, -3.81595) -> (-97, -3.81595)
  line L35 (-97, -3.81595) -> (-97, -48.81595)
  line L36 (82.5, 30) -> (-82.5, 30)
  line L37 (-82.5, 30) -> (-82.5, 55)
  line L38 (-82.5, 55) -> (82.5, 55)
  line L39 (82.5, 55) -> (82.5, 30)
  point P0 (0, 30)
  constraint horizontal L36
  constraint vertical L37
  constraint horizontal L38
  constraint vertical L39
  constraint midpoint L36 P0
  constraint vertical origin P0
extrude "Extrusion29" cut sketch "Skizze28" against normal blind 12 contours L36 L37 L38 L39 picked at (27.5, 38.333333) bodies 6
sketch "Skizze29" plane through (0, 0, 63) normal (0, 0, 1) x (-1, 0, 0)
  line L0 (-82.5, 30) -> (-82.5, 55)
  line L1 (-82.5, 55) -> (82.5, 55)
  line L2 (82.5, 55) -> (82.5, 30)
  line L3 (82.5, 30) -> (-82.5, 30)
  circle A0 centre (80, 0) radius 4
  circle A1 centre (60, 0) radius 4
  circle A2 centre (60, -25) radius 6
  circle A3 centre (40, -25) radius 6
  circle A4 centre (80, -25) radius 6
  line L4 (-66.616861, -35.006887) -> (-66.616861, -15.006887)
  line L5 (-66.616861, -15.006887) -> (-53.616861, -15.006887)
  line L6 (-53.616861, -15.006887) -> (-53.616861, -35.006887)
  line L7 (-53.616861, -35.006887) -> (-66.616861, -35.006887)
  line L8 (-86.409655, -35.161049) -> (-86.409655, -15.161049)
  line L9 (-86.409655, -15.161049) -> (-73.409655, -15.161049)
  line L10 (-73.409655, -15.161049) -> (-73.409655, -35.161049)
  line L11 (-73.409655, -35.161049) -> (-86.409655, -35.161049)
  circle A5 centre (-60, -50) radius 3
  circle A6 centre (-80, -50) radius 3
  circle A7 centre (80, -50) radius 6
  circle A8 centre (60, -50) radius 6
  circle A9 centre (40.782868, -50.075086) radius 6
  line L12 (-97, -48.81595) -> (-100, -48.81595)
  line L13 (-100, -48.81595) -> (-100, -58.81595)
  line L14 (-100, -58.81595) -> (-97, -58.81595)
  line L15 (-97, -58.81595) -> (-97, -70)
  line L16 (-97, -70) -> (97, -70)
  line L17 (97, -70) -> (97, -63.742894)
  line L18 (97, -63.742894) -> (100, -63.742894)
  line L19 (100, -63.742894) -> (100, -53.742894)
  line L20 (100, -53.742894) -> (97, -53.742894)
  line L21 (97, -53.742894) -> (97, -6.242894)
  line L22 (97, -6.242894) -> (100, -6.242894)
  line L23 (100, -6.242894) -> (100, 3.757106)
  line L24 (100, 3.757106) -> (97, 3.757106)
  line L25 (97, 3.757106) -> (97, 51.257106)
  line L26 (97, 51.257106) -> (100, 51.257106)
  line L27 (100, 51.257106) -> (100, 61.257106)
  line L28 (100, 61.257106) -> (97, 61.257106)
  line L29 (97, 61.257106) -> (97, 70)
  line L30 (97, 70) -> (-97, 70)
  line L31 (-97, 70) -> (-97, 61.18405)
  line L32 (-97, 61.18405) -> (-100, 61.18405)
  line L33 (-100, 61.18405) -> (-100, 51.18405)
  line L34 (-100, 51.18405) -> (-97, 51.18405)
  line L35 (-97, 51.18405) -> (-97, 6.18405)
  line L36 (-97, 6.18405) -> (-100, 6.18405)
  line L37 (-100, 6.18405) -> (-100, -3.81595)
  line L38 (-100, -3.81595) -> (-97, -3.81595)
  line L39 (-97, -3.81595) -> (-97, -48.81595)
sketch "Skizze31" plane through (0, -70, 0) normal (0, -1, 0) x (1, 0, 0)
  line L0 (97, 60) -> (-97, 60)
  line L1 (-97, 60) -> (-97, 57.564108)
  line L2 (-97, 57.564108) -> (-100, 57.564108)
  line L3 (-100, 57.564108) -> (-100, 47.564108)
  line L4 (-100, 47.564108) -> (-97, 47.564108)
  line L5 (-97, 47.564108) -> (-97, 37.564108)
  line L6 (-97, 37.564108) -> (-100, 37.564108)
  line L7 (-100, 37.564108) -> (-100, 27.564108)
  line L8 (-100, 27.564108) -> (-97, 27.564108)
  line L9 (-97, 27.564108) -> (-97, 17.564108)
  line L10 (-97, 17.564108) -> (-100, 17.564108)
  line L11 (-100, 17.564108) -> (-100, 7.564108)
  line L12 (-100, 7.564108) -> (-97, 7.564108)
  line L13 (-97, 7.564108) -> (-97, 3)
  line L14 (-97, 3) -> (-86.937173, 3)
  line L15 (-86.937173, 3) -> (-86.937173, 0)
  line L16 (-86.937173, 0) -> (-76.937173, 0)
  line L17 (-76.937173, 0) -> (-76.937173, 3)
  line L18 (-76.937173, 3) -> (-31.937173, 3)
  line L19 (-31.937173, 3) -> (-31.937173, 0)
  line L20 (-31.937173, 0) -> (-21.937173, 0)
  line L21 (-21.937173, 0) -> (-21.937173, 3)
  line L22 (-21.937173, 3) -> (23.062827, 3)
  line L23 (23.062827, 3) -> (23.062827, 0)
  line L24 (23.062827, 0) -> (33.062827, 0)
  line L25 (33.062827, 0) -> (33.062827, 3)
  line L26 (33.062827, 3) -> (78.062827, 3)
  line L27 (78.062827, 3) -> (78.062827, 0)
  line L28 (78.062827, 0) -> (88.062827, 0)
  line L29 (88.062827, 0) -> (88.062827, 3)
  line L30 (88.062827, 3) -> (97.000001, 3)
  line L31 (97.000001, 3) -> (97.000001, 7.960939)
  line L32 (97.000001, 7.960939) -> (100.000001, 7.960939)
  line L33 (100.000001, 7.960939) -> (100.000001, 17.960939)
  line L34 (100.000001, 17.960939) -> (97.000001, 17.960939)
  line L35 (97.000001, 17.960939) -> (97.000001, 27.960939)
  line L36 (97.000001, 27.960939) -> (100.000001, 27.960939)
  line L37 (100.000001, 27.960939) -> (100.000001, 37.960939)
  line L38 (100.000001, 37.960939) -> (97.000001, 37.960939)
  line L39 (97.000001, 37.960939) -> (97.000001, 47.960939)
  line L40 (97.000001, 47.960939) -> (100.000001, 47.960939)
  line L41 (100.000001, 47.960939) -> (100.000001, 57.960939)
  line L42 (100.000001, 57.960939) -> (97.000001, 57.960939)
  line L43 (97.000001, 57.960939) -> (97, 60)
sketch "Skizze32" plane through (-100, 0, 0) normal (-1, 0, 0) x (0, -1, 0)
  line L0 (61.257106, 63) -> (61.257106, 60)
  line L1 (61.257106, 60) -> (51.257106, 60)
  line L2 (51.257106, 60) -> (51.257106, 63)
  line L3 (51.257106, 63) -> (3.757106, 63)
  line L4 (3.757106, 63) -> (3.757106, 60)
  line L5 (3.757106, 60) -> (-6.242894, 60)
  line L6 (-6.242894, 60) -> (-6.242894, 63)
  line L7 (-6.242894, 63) -> (-53.742894, 63)
  line L8 (-53.742894, 63) -> (-53.742894, 60)
  line L9 (-53.742894, 60) -> (-63.742894, 60)
  line L10 (-63.742894, 60) -> (-63.742894, 63)
  line L11 (-63.742894, 63) -> (-70, 63)
  line L12 (-70, 63) -> (-70, 58.048511)
  line L13 (-70, 58.048511) -> (-67, 58.048511)
  line L14 (-67, 58.048511) -> (-67, 48.048511)
  line L15 (-67, 48.048511) -> (-70, 48.048511)
  line L16 (-70, 48.048511) -> (-70, 38.048511)
  line L17 (-70, 38.048511) -> (-67, 38.048511)
  line L18 (-67, 38.048511) -> (-67, 28.048511)
  line L19 (-67, 28.048511) -> (-70, 28.048511)
  line L20 (-70, 28.048511) -> (-70, 18.048511)
  line L21 (-70, 18.048511) -> (-67, 18.048511)
  line L22 (-67, 18.048511) -> (-67, 8.048511)
  line L23 (-67, 8.048511) -> (-70, 8.048511)
  line L24 (-70, 8.048511) -> (-70, 3)
  line L25 (-70, 3) -> (-60, 3)
  line L26 (-60, 3) -> (-60, 0)
  line L27 (-60, 0) -> (-50, 0)
  line L28 (-50, 0) -> (-50, 3)
  line L29 (-50, 3) -> (-23.333333, 3)
  line L30 (-23.333333, 3) -> (-23.333333, 0)
  line L31 (-23.333333, 0) -> (-13.333333, 0)
  line L32 (-13.333333, 0) -> (-13.333333, 3)
  line L33 (-13.333333, 3) -> (13.333333, 3)
  line L34 (13.333333, 3) -> (13.333333, 0)
  line L35 (13.333333, 0) -> (23.333333, 0)
  line L36 (23.333333, 0) -> (23.333333, 3)
  line L37 (23.333333, 3) -> (50, 3)
  line L38 (50, 3) -> (50, 0)
  line L39 (50, 0) -> (60, 0)
  line L40 (60, 0) -> (60, 3)
  line L41 (60, 3) -> (70, 3)
  line L42 (70, 3) -> (70, 7.564108)
  line L43 (70, 7.564108) -> (67, 7.564108)
  line L44 (67, 7.564108) -> (67, 17.564108)
  line L45 (67, 17.564108) -> (70, 17.564108)
  line L46 (70, 17.564108) -> (70, 27.564108)
  line L47 (70, 27.564108) -> (67, 27.564108)
  line L48 (67, 27.564108) -> (67, 37.564108)
  line L49 (67, 37.564108) -> (70, 37.564108)
  line L50 (70, 37.564108) -> (70, 47.564108)
  line L51 (70, 47.564108) -> (67, 47.564108)
  line L52 (67, 47.564108) -> (67, 57.564108)
  line L53 (67, 57.564108) -> (70, 57.564108)
  line L54 (70, 57.564108) -> (70, 63)
  line L55 (70, 63) -> (61.257106, 63)
sketch "Skizze33" plane through (100, 0, 0) normal (1, 0, 0) x (0, 1, 0)
  line L0 (58.81595, 63) -> (58.81595, 60)
  line L1 (58.81595, 60) -> (48.81595, 60)
  line L2 (48.81595, 60) -> (48.81595, 63)
  line L3 (48.81595, 63) -> (3.81595, 63)
  line L4 (3.81595, 63) -> (3.81595, 60)
  line L5 (3.81595, 60) -> (-6.18405, 60)
  line L6 (-6.18405, 60) -> (-6.18405, 63)
  line L7 (-6.18405, 63) -> (-51.18405, 63)
  line L8 (-51.18405, 63) -> (-51.18405, 60)
  line L9 (-51.18405, 60) -> (-61.18405, 60)
  line L10 (-61.18405, 60) -> (-61.18405, 63)
  line L11 (-61.18405, 63) -> (-70, 63)
  line L12 (-70, 63) -> (-70, 57.960939)
  line L13 (-70, 57.960939) -> (-67, 57.960939)
  line L14 (-67, 57.960939) -> (-67, 47.960939)
  line L15 (-67, 47.960939) -> (-70, 47.960939)
  line L16 (-70, 47.960939) -> (-70, 37.960939)
  line L17 (-70, 37.960939) -> (-67, 37.960939)
  line L18 (-67, 37.960939) -> (-67, 27.960939)
  line L19 (-67, 27.960939) -> (-70, 27.960939)
  line L20 (-70, 27.960939) -> (-70, 17.960939)
  line L21 (-70, 17.960939) -> (-67, 17.960939)
  line L22 (-67, 17.960939) -> (-67, 7.960939)
  line L23 (-67, 7.960939) -> (-70, 7.960939)
  line L24 (-70, 7.960939) -> (-70, 3)
  line L25 (-70, 3) -> (-58.902439, 3)
  line L26 (-58.902439, 3) -> (-58.902439, 0)
  line L27 (-58.902439, 0) -> (-48.902439, 0)
  line L28 (-48.902439, 0) -> (-48.902439, 3)
  line L29 (-48.902439, 3) -> (-22.235772, 3)
  line L30 (-22.235772, 3) -> (-22.235772, 0)
  line L31 (-22.235772, 0) -> (-12.235772, 0)
  line L32 (-12.235772, 0) -> (-12.235772, 3)
  line L33 (-12.235772, 3) -> (14.430895, 3)
  line L34 (14.430895, 3) -> (14.430895, 0)
  line L35 (14.430895, 0) -> (24.430895, 0)
  line L36 (24.430895, 0) -> (24.430895, 3)
  line L37 (24.430895, 3) -> (51.097561, 3)
  line L38 (51.097561, 3) -> (51.097561, 0)
  line L39 (51.097561, 0) -> (61.097561, 0)
  line L40 (61.097561, 0) -> (61.097561, 3)
  line L41 (61.097561, 3) -> (70, 3)
  line L42 (70, 3) -> (70, 6.682652)
  line L43 (70, 6.682652) -> (67, 6.682652)
  line L44 (67, 6.682652) -> (67, 16.682652)
  line L45 (67, 16.682652) -> (70, 16.682652)
  line L46 (70, 16.682652) -> (70, 27.682652)
  line L47 (70, 27.682652) -> (67, 27.682652)
  line L48 (67, 27.682652) -> (67, 37.682652)
  line L49 (67, 37.682652) -> (70, 37.682652)
  line L50 (70, 37.682652) -> (70, 48.682652)
  line L51 (70, 48.682652) -> (67, 48.682652)
  line L52 (67, 48.682652) -> (67, 58.682652)
  line L53 (67, 58.682652) -> (70, 58.682652)
  line L54 (70, 58.682652) -> (70, 63)
  line L55 (70, 63) -> (58.81595, 63)
sketch "Skizze34" plane through (0, 70, 0) normal (0, 1, 0) x (-1, 0, 0)
  line L0 (97, 63) -> (97, 60)
  line L1 (97, 60) -> (-96.999959, 60)
  line L2 (-96.999959, 60) -> (-96.999959, 58.682652)
  line L3 (-96.999959, 58.682652) -> (-100.099959, 58.682652)
  line L4 (-100.099959, 58.682652) -> (-100.099959, 48.682652)
  line L5 (-100.099959, 48.682652) -> (-96.999959, 48.682652)
  line L6 (-96.999959, 48.682652) -> (-96.999959, 37.682652)
  line L7 (-96.999959, 37.682652) -> (-100.099959, 37.682652)
  line L8 (-100.099959, 37.682652) -> (-100.099959, 27.682652)
  line L9 (-100.099959, 27.682652) -> (-96.999959, 27.682652)
  line L10 (-96.999959, 27.682652) -> (-96.999959, 16.682652)
  line L11 (-96.999959, 16.682652) -> (-100.099959, 16.682652)
  line L12 (-100.099959, 16.682652) -> (-100.099959, 6.682652)
  line L13 (-100.099959, 6.682652) -> (-96.999959, 6.682652)
  line L14 (-96.999959, 6.682652) -> (-96.999959, 3)
  line L15 (-96.999959, 3) -> (-89.745041, 3)
  line L16 (-89.745041, 3) -> (-89.745041, 0)
  line L17 (-89.745041, 0) -> (-79.745041, 0)
  line L18 (-79.745041, 0) -> (-79.745041, 3)
  line L19 (-79.745041, 3) -> (-33.078374, 3)
  line L20 (-33.078374, 3) -> (-33.078374, 0)
  line L21 (-33.078374, 0) -> (-23.078374, 0)
  line L22 (-23.078374, 0) -> (-23.078374, 3)
  line L23 (-23.078374, 3) -> (23.588293, 3)
  line L24 (23.588293, 3) -> (23.588293, 0)
  line L25 (23.588293, 0) -> (33.588293, 0)
  line L26 (33.588293, 0) -> (33.588293, 3)
  line L27 (33.588293, 3) -> (80.254959, 3)
  line L28 (80.254959, 3) -> (80.254959, 0)
  line L29 (80.254959, 0) -> (90.254959, 0)
  line L30 (90.254959, 0) -> (90.254959, 3)
  line L31 (90.254959, 3) -> (97.000041, 3)
  line L32 (97.000041, 3) -> (97.000041, 8.048511)
  line L33 (97.000041, 8.048511) -> (100.000041, 8.048511)
  line L34 (100.000041, 8.048511) -> (100.000041, 18.048511)
  line L35 (100.000041, 18.048511) -> (97.000041, 18.048511)
  line L36 (97.000041, 18.048511) -> (97.000041, 28.048511)
  line L37 (97.000041, 28.048511) -> (100.000041, 28.048511)
  line L38 (100.000041, 28.048511) -> (100.000041, 38.048511)
  line L39 (100.000041, 38.048511) -> (97.000041, 38.048511)
  line L40 (97.000041, 38.048511) -> (97.000041, 48.048511)
  line L41 (97.000041, 48.048511) -> (100.000041, 48.048511)
  line L42 (100.000041, 48.048511) -> (100.000041, 58.048511)
  line L43 (100.000041, 58.048511) -> (97.000041, 58.048511)
  line L44 (97.000041, 58.048511) -> (97.000041, 63)
  line L45 (97.000041, 63) -> (97, 63)